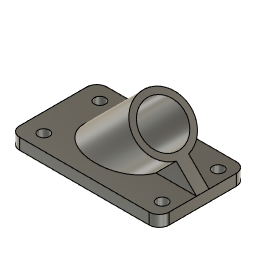
Day #11 v1 (Autodesk Fusion 360 design; units mm, degrees)
Autodesk Fusion 360 part; units mm, degrees
note: some values were not read from the file. Chosen so that the rebuilt part matches the saved one: where a step ends. Set by a fixed rule: which sketch regions a step uses.
sketch "Sketch1" plane through (0, 0, 0) normal (0, 0, 1) x (1, 0, 0)
  line L0 (57.5726, 35) -> (-62.4274, 35)
  line L1 (-62.4274, 35) -> (-62.4274, -35)
  line L2 (-62.4274, -35) -> (57.5726, -35)
  line L3 (57.5726, -35) -> (57.5726, 35)
  line L4 (57.5726, 35) -> (-62.4274, -35) construction
  line L5 (-62.4274, 35) -> (57.5726, -35) construction
  point P0 (-2.4274, 0)
  dimension "d1" = 120
  dimension "d2" = 70
  constraint horizontal L0
  constraint perpendicular L0 L1
  constraint parallel L0 L2
  constraint parallel L1 L3
  constraint coincident L4 P0
  constraint coincident L5 P0
  measures "d1" distance of L1.end L2.end
  measures "d2" distance of L0.end L1.end
extrude "Extrude1" add sketch "Sketch1" along normal blind 9
ref_plane "WorkPlane1" through (0, 12.125, 0) normal (0.707107, 0, 0.707107) x (0, 1, 0)
ref_plane "WorkPlane2" through (33.2863, 12.125, 33.2863) normal (0.707107, 0, 0.707107) x (0, 1, 0)
sketch "Sketch2" plane through (33.2863, 0, 33.2863) normal (0.707107, 0, 0.707107) x (0, 1, 0)
  circle A0 centre (0, 10.654) radius 22.5
  line L0 (0, -1.2374) -> (0, -15.9099)
  line L1 (-35, -34.346) -> (35, -34.346)
  line L2 (-5, 10) -> (-5, -34.346)
  line L3 (-5, -34.346) -> (5, -34.346)
  line L4 (5, -34.346) -> (5, 10)
  line L5 (5, 10) -> (-5, 10)
  dimension "d7" = 45
  dimension "d8" = 45
  dimension "d9" = 10
  constraint coincident A0.centre L0
  constraint perpendicular L2 L3
  constraint parallel L2 L4
  constraint parallel L3 L5
  constraint coincident L1 L2.end
  constraint perpendicular L1 L2
  measures "d7" diameter of A0
  measures "d8" distance of A0.centre L1
  measures "d9" distance of L2.end L3.end
extrude "Extrude2" add sketch "Sketch2" along normal up to far side of body 1
hole "Hole1" at (25.7528, 0, 40.8198) direction (-0.707107, 0, -0.707107) diameter 35 end through all
sketch "Sketch3" plane through (0, 0, 9) normal (0, 0, 1) x (-1, 0, 0)
  line L0 (-24.9572, -5) -> (-57.5726, -5)
  line L1 (-57.5726, -5) -> (-57.5726, -35)
  line L2 (-57.5726, -35) -> (62.4274, -35)
  line L3 (62.4274, -35) -> (62.4274, 35)
  line L4 (62.4274, 35) -> (-57.5726, 35)
  line L5 (-57.5726, 35) -> (-57.5726, 5)
  line L6 (-57.5726, 5) -> (-24.9572, 5)
  ellipse E0 centre (6.067, 0) end of major axis (-25.7528, 0) minor radius 22.5 (-24.9572, -5) -> (-24.9572, 5) ccw
  line L7 (47.5, -22.5) -> (-47.5, -22.5)
  line L8 (-47.5, -22.5) -> (-47.5, 22.5)
  line L9 (-47.5, 22.5) -> (47.5, 22.5)
  line L10 (47.5, 22.5) -> (47.5, -22.5)
  line L11 (47.5, -22.5) -> (-47.5, 22.5) construction
  line L12 (-47.5, -22.5) -> (47.5, 22.5) construction
  dimension "d13" = 95
  dimension "d14" = 45
  constraint horizontal L7
  constraint perpendicular L7 L8
  constraint parallel L7 L9
  constraint parallel L8 L10
  constraint coincident L11 origin
  constraint coincident L12 origin
  measures "d13" distance of L8.end L9.end
  measures "d14" distance of L7.end L8.end
hole "Hole2" at (-47.5, 22.5, 9) at (-47.5, -22.5, 9) at (47.5, 22.5, 9) at (47.5, -22.5, 9) direction (0, 0, -1) diameter 9 end through all
fillet "Fillet1" radius 8 4 edges at (57.5726, 35, 4.5) (57.5726, -35, 4.5) (-62.4274, 35, 4.5) (-62.4274, -35, 4.5)
